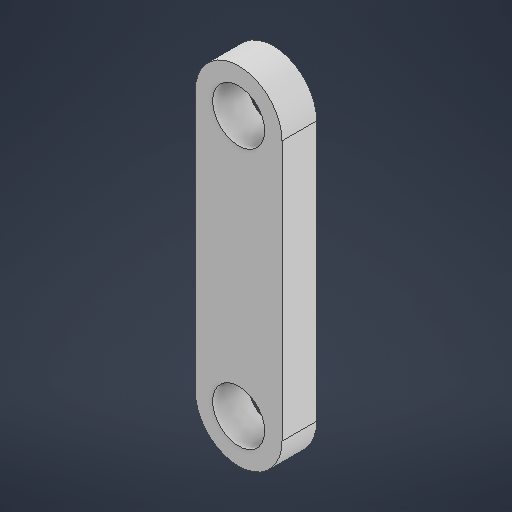
# Autodesk Inventor part: 连杆2
Saved by Autodesk Inventor 2025 (Build 290162000, 162)
## iProperties
Created: 2026-04-24
Part Number: 连杆2
Material: 常规
Document SubType Name: Modeling
Designer: XH
Density: 1 g/cm^3
Appearance: 默认
Author: XH
Autodesk Inventor part; units mm, degrees
ref_plane "YZ Plane" through (0, 0, 0) normal (1, 0, 0) x (0, 1, 0)
ref_plane "XZ Plane" through (0, 0, 0) normal (0, 1, 0) x (-1, 0, 0)
ref_plane "XY Plane" through (0, 0, 0) normal (0, 0, 1) x (1, 0, 0)
sketch "草图1" plane through (0, 0, 0) normal (0, 0, 1) x (1, 0, 0)
  line L0 (0, 0) -> (0, 15) construction
  line L1 (2.5, 0) -> (2.5, 15)
  line L2 (-2.5, 15) -> (-2.5, 0)
  arc A0 (-2.5, 0) -> (2.5, 0) centre (0, 0) ccw
  arc A1 (2.5, 15) -> (-2.5, 15) centre (0, 15) ccw
  point P0 (0, 7.5)
  point P1 (0, -2.5)
  point P2 (0, 17.5)
  dimension "d2" = 20
  dimension "d3" = 5
  constraints: 8 end point, 6 point on circle, 4 tangent, 2 centre point, 1 midpoint, 1 parallel, 1 vertical
  measures "d2" distance of point (0, -2.5) point (0, 17.5)
  measures "d3" distance between parallel lines of L2 L1
extrude "拉伸1" add sketch "草图1" along normal blind 2
sketch "草图2" plane through (0, 0, 2) normal (0, 0, 1) x (1, 0, 0)
  circle A0 centre (0, 0) radius 1.5
  arc A1 (2.5, 15) -> (-2.5, 15) centre (0, 15) ccw projected
  circle A2 centre (0, 15) radius 1.5
  dimension "d4" = 3
  dimension "d5" = 3
  constraints: 2 centre point, 2 coincident
  measures "d4" diameter of A0
  measures "d5" diameter of A2
extrude "拉伸2" cut sketch "草图2" against normal blind 3
